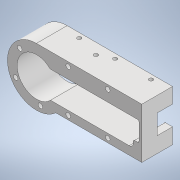
# Autodesk Inventor part: Mech Panel v7 infill_01
Saved by Autodesk Inventor 2022 (Build 260153000, 153)
## iProperties
Created: 2022-09-24
Part Number: Mech Panel v7 infill_01
Material: Generic
Document SubType Name: Modeling
Designer: matt
Density: 1 g/cm^3
Appearance: Default
Author: matt
Autodesk Inventor part; units mm, degrees
sketch "Sketch1" plane through (0, 0, 0) normal (0, 0, 1) x (1, 0, 0)
  circle A0 centre (0, 0) radius 11.1125 construction
  line L0 (104.364, -18.65) -> (70.364, -18.65) construction
  line L1 (104.364, 18.65) -> (70.364, 18.65) construction
  line L2 (23.9529, -7.067) -> (23.9529, 14.933) construction
  arc A1 (-39, 0) -> (23.4665, -31.15) centre (0, 0) ccw construction
  line L3 (50.614, 19.35) -> (60.114, 19.35) construction
  line L4 (50.614, 19.85) -> (60.114, 19.85)
  line L5 (60.114, -18.65) -> (50.614, -18.65) construction
  arc A2 (19.7478, 19.85) -> (20.4274, -19.15) centre (0, 0) ccw
  line L6 (0, 42) -> (171.45, 42)
  line L7 (-238.861, -48) -> (171.45, -48) construction
  line L8 (-39, 0) -> (-42, 0) construction
  arc A3 (0, 42) -> (28.1723, -31.15) centre (0, 0) ccw
  circle A4 centre (0, 0) radius 14.224
  line L9 (171.45, 42) -> (171.45, -31.15)
  line L10 (19.7478, 19.85) -> (152.6937, 19.85)
  line L11 (152.6937, -19.15) -> (20.4274, -19.15)
  line L12 (23.4665, -31.15) -> (171.45, -31.15)
  line L13 (0, 28) -> (0, 30)
  line L14 (0, 30) -> (117.475, 30)
  line L15 (142.2077, -8.6311) -> (152.6937, -8.6311)
  line L16 (117.475, 30) -> (117.475, 19.85) construction
  line L17 (117.475, -19.15) -> (117.475, -31.15)
  line L18 (140.3854, -10.4534) -> (140.3854, -13.15)
  line L19 (148.6937, 19.85) -> (148.6937, -6.6311)
  line L20 (117.475, 30) -> (171.45, 30) construction
  line L21 (-34.4683, 6.0777) -> (0, 0) construction
  line L22 (-22.4976, -26.8116) -> (0, 0) construction
  line L23 (0, 0) -> (11.9707, -32.8892) construction
  circle A5 centre (0, 0) radius 34 construction
  line L24 (117.475, 19.85) -> (148.6937, 19.85)
  line L25 (148.6937, 19.85) -> (148.6937, 30)
  line L26 (152.6937, 30) -> (117.475, 30)
  line L27 (117.475, 30) -> (117.475, 19.85) construction
  line L28 (34.114, 20.2591) -> (34.114, 32) construction
  line L29 (65.364, 20.2591) -> (65.364, 32) construction
  line L30 (33.864, 19.85) -> (33.864, 32) construction
  line L31 (65.614, 19.85) -> (65.614, 32) construction
  line L32 (22.4976, 36) -> (171.45, 36) construction
  line L33 (171.45, -25.15) -> (28.0371, -25.15) construction
  circle A6 centre (-24.2686, 23.8125) radius 3.35
  circle A7 centre (-30.1464, -15.7223) radius 3.35
  circle A8 centre (5.6371, -33.5294) radius 3.35
  circle A9 centre (33.6303, -5) radius 3.35
  circle A10 centre (15.1476, 30.4393) radius 3.35
  circle A11 centre (46.0375, 36) radius 3.35
  circle A12 centre (46.0375, -25.15) radius 3.35
  circle A13 centre (136.0375, 36) radius 3.35
  circle A14 centre (136.0375, -25.15) radius 3.35
  arc A15 (146.6937, -8.6311) -> (148.6937, -6.6311) centre (146.6937, -6.6311) ccw
  arc A16 (142.2077, -8.6311) -> (140.3854, -10.4534) centre (142.2077, -10.4534) ccw
  arc A17 (148.6937, 28) -> (146.6937, 30) centre (146.6937, 28) ccw
  line L34 (152.6937, 42) -> (152.6937, -31.15)
  line L35 (148.6937, 11.5374) -> (171.45, 11.5374)
  line L36 (171.45, 11.5374) -> (171.45, -8.6311)
  line L37 (171.45, -8.6311) -> (152.6937, -8.6311)
  line L38 (148.6937, -8.6435) -> (148.6937, 11.5374)
  circle A18 centre (103.364, 36) radius 3.35
  circle A19 centre (103.364, -25.15) radius 3.35
  line L39 (140.3854, -10.4534) -> (140.3854, -0.553)
  line L40 (142.3854, 1.447) -> (148.6937, 1.447)
  arc A20 (142.3854, 1.447) -> (140.3854, -0.553) centre (142.3854, -0.553) ccw
  arc A21 (134.3854, -19.15) -> (140.3854, -13.15) centre (134.3854, -13.15) ccw
  line L41 (140.747, -6.35) -> (140.747, 7.9375) construction
  arc A22 (148.6937, 17.85) -> (146.6937, 19.85) centre (146.6937, 17.85) ccw
  arc A23 (146.6937, 19.85) -> (148.6937, 21.85) centre (146.6937, 21.85) ccw
  point P0 (171.45, -22)
  point P1 (140.3854, -8.6311)
  point P2 (171.45, -7.65)
  point P3 (171.45, 7)
  point P4 (148.6937, -8.6311)
  point P5 (33.864, 30)
  point P6 (65.614, 30)
  point P7 (140.2077, 19.85)
  point P8 (148.6937, 17.7587)
  point P9 (152.6937, 11.5374)
  point P10 (152.6937, -8.6435)
  point P11 (148.6937, -8.6311)
  dimension "d38" = 68
  dimension "d0" = 78
  dimension "d4" = 0.5
  dimension "d6" = 56
  dimension "d8" = 90
  dimension "d9" = 28.448
  dimension "d12" = 12
  dimension "d23" = 12
  dimension "d24" = 0.5
  dimension "d25" = 38
  dimension "d27" = 42
  dimension "d33" = 80
  dimension "d36" = 39
  dimension "d37" = 28
  dimension "d39" = 6
  dimension "d49" = 0.25
  dimension "d50" = 0.25
  dimension "d55" = 6
  dimension "d56" = 6.7
  dimension "d59" = 360
  dimension "d62" = 6.7
  dimension "d65" = 90
  dimension "d70" = 171.45
  dimension "d84" = 2
  dimension "d92" = 4
  dimension "d102" = 2
  dimension "d111" = 6
  dimension "d116" = 4
  dimension "d117" = 2
  constraints: 82 end point, 34 point on line, 23 centre point, 22 point on circle, 14 tangent, 12 horizontal, 10 parallel, 9 perpendicular, 6 coincident, 4 vertical, 3 collinear, 1 midpoint, 40 other
  measures "d0" diameter of A1
  measures "d4" distance between parallel lines of L3 L4
  measures "d6" diameter of A2
  measures "d8" distance between parallel lines of L7 L6
  measures "d9" diameter of A4
  measures "d12" distance between parallel lines of L14 L6
  measures "d23" distance between parallel lines of L12 L11
  measures "d24" distance between parallel lines of L11 L5
  measures "d25" distance between parallel lines of L5 L3
  measures "d27" radius of A3
  measures "d33" angle of L2 L21
  measures "d36" radius of A1
  measures "d37" radius of A2
  measures "d39" distance from line of L6 L32.start
  measures "d49" distance between parallel lines of L28 L30
  measures "d50" distance between parallel lines of L29 L31
  measures "d55" distance between parallel lines of L12 L33
  measures "d56" diameter of A6
  measures "d62" diameter of A11
  measures "d65" distance of A11.centre A13.centre
  measures "d84" radius of A17
  measures "d92" distance between parallel lines of L34 L19
  measures "d102" radius of A20
  measures "d111" radius of A21
  measures "d116" diameter of A22
  measures "d117" radius of A23
extrude "Extrusion1" add sketch "Sketch1" along normal blind 28.448 contours A2 L11 L17 L12 A3 L6 L34 L26 L14 A10 L13 | L25 L26 L34 L10 | L11 L34 L12 L17 | A10 L14 | A21 L18 A16 L15 L34 L11 | A13 | A14 picked at (15.3429, 31.3449)
extrude "Extrusion2" add sketch "Sketch1" along normal blind 16.1 from surface at 28.448 contours L10 A2 L13 L14 A10 L26 A17 L25 A23 L4 | A2 L11 L17 L12 A3 L6 L34 L26 L14 A10 L13 | A23 L25 L10 | L25 L26 L34 L10 | L11 L34 L12 L17 | A10 L14 | L14 A10 | A17 L26 L25 | A21 L18 A16 L15 L34 L11 | A13 | A14
sketch "Sketch2" plane through (0, 42, 0) normal (0, 1, 0) x (1, 0, 0)
  circle A0 centre (24.3468, -37.648) radius 2.8
  line L0 (171.45, -43.548) -> (0, -43.548) construction
  line L1 (152.6937, 0) -> (0, 0) projected
  line L2 (0, 0) -> (0, -44.548) projected
  line L3 (0, -44.548) -> (152.6937, -44.548) projected
  line L4 (152.6937, 0) -> (152.6937, -44.548) projected
  circle A1 centre (76.3468, -37.648) radius 2.8
  circle A2 centre (128.3468, -37.648) radius 2.8
  line L5 (152.6937, 0) -> (152.6937, -44.548) construction
  line L6 (152.6937, -22.274) -> (0, -22.274) construction
  line L7 (0, 0) -> (0, -28.448) construction
  circle A3 centre (24.3468, -6.9) radius 2.8
  circle A4 centre (76.3468, -6.9) radius 2.8
  circle A5 centre (128.3468, -6.9) radius 2.8
  circle A6 centre (57.6393, -16.071) radius 3
  dimension "d73" = 5.6
  dimension "d93" = 24.3468
  dimension "d94" = 152.6937
  dimension "d97" = 52
  dimension "d108" = 6.9
  constraints: 7 centre point, 3 symmetric about line, 2 end point, 1 horizontal, 1 midpoint, 1 perpendicular, 1 point on line, 7 other
  measures "d73" diameter of A0
  measures "d93" distance from line of L2 A0.centre
  measures "d94" distance between parallel lines of L4 L2
  measures "d97" distance of A0.centre A1.centre
  measures "d108" distance from line of L3 A0.centre
extrude "Extrusion4" cut sketch "Sketch2" against normal blind 15.1 contours A3 | A4 | A5 | A6
ref_plane "Work Plane1" through (0, 0, 12) normal (0, 0, -1) x (-1, 0, 0)
sketch "Sketch6" plane through (152.6937, -31.15, 0) normal (1, 0, 0) x (0, 0, -1)
  line L0 (0, 30.597) -> (-28.448, 30.597)
  circle A0 centre (-7.9375, 30.597) radius 3
  dimension "d104" = 6
  constraints: 2 end point, 1 centre point, 1 point on line
  measures "d104" diameter of A0
ref_plane "Work Plane2" through (-23.5188, -31.15, 0) normal (1, 0, 0) x (0, 0, -1)
extrude "Extrusion6" cut sketch "Sketch6" against normal blind 30 from surface at -176.2125
extrude "Extrusion7" add sketch "Sketch1" against normal blind 15.1 from surface at 28.448 contours L10 A2 L13 L14 A10 L26 A17 L25 A23 L4 | A23 L25 L10 | L14 A10 | A17 L26 L25 picked at (15.3464, 28.8029)
ref_plane "Work Plane3" through (0, 0, 22.274) normal (0, 0, -1) x (-1, 0, 0)
extrude "Extrusion8" add sketch "Sketch1" along normal up to surface (22.274 mm away) from surface at 22.274 contours L10 L19 A22 | L25 L26 L34 L10 | L10 L34 L35 L19 | L35 L34 L15 L38 L19 | A17 L26 L25 | L38 L15 A15
equation "\"d12\" = d23"
equation "\"d10\" = d9"
body "Solid1"
